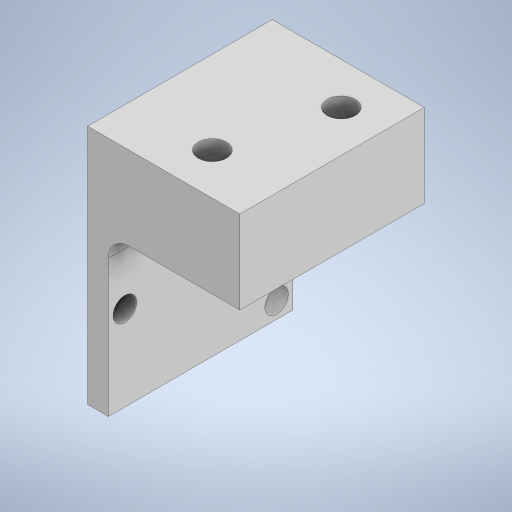
# Autodesk Inventor part: Limit Switch Top V1
Saved by Autodesk Inventor 2024.2 (Build 282272000, 272)
## iProperties
Created: 2024-08-22
Part Number: Limit Switch Top V1
Material: Generic
Document SubType Name: Modeling
Designer: balmo
Density: 1 g/cm^3
Appearance: Default
Author: balmo
## iProperties of the stored document Limit Switch Top V1_3DPrint.ipt
Created: 2024-08-22
Part Number: Limit Switch Top V1_3DPrint
Material: Generic
Document SubType Name: Modeling
Designer: balmo
Density: 1 g/cm^3
Appearance: Default
Author: balmo
Autodesk Inventor part; units mm, degrees
ref_plane "YZ Plane" through (0, 0, 0) normal (1, 0, 0) x (0, 1, 0)
ref_plane "XZ Plane" through (0, 0, 0) normal (0, 1, 0) x (-1, 0, 0)
ref_plane "XY Plane" through (0, 0, 0) normal (0, 0, 1) x (1, 0, 0)
sketch "Sketch1" plane through (0, 0, 0) normal (0, 0, 1) x (1, 0, 0)
  line L0 (0, 0) -> (3.175, 0)
  line L1 (3.175, 0) -> (3.175, 24.13)
  line L2 (0, 36.83) -> (0, 0)
  line L3 (23.2455, 36.83) -> (23.2455, 24.13)
  line L4 (23.2455, 24.13) -> (3.175, 24.13)
  line L5 (0, 36.83) -> (23.2455, 36.83)
  dimension "d0" = 12.7
  dimension "d1" = 3.175
  dimension "d2" = 36.83
  constraints: 12 end point, 2 horizontal, 1 parallel, 1 perpendicular
  measures "d0" distance between parallel lines of L4 L5
  measures "d1" distance between parallel lines of L2 L1
  measures "d2" distance between parallel lines of L5 L0
extrude "Extrusion1" add sketch "Sketch1" along normal blind 28.194
sketch "Sketch2" plane through (3.175, 0, 0) normal (1, 0, 0) x (0, 0, -1)
  circle A0 centre (-2.5, 2.5) radius 1.8
  circle A1 centre (-25.694, 13) radius 1.8
  line L0 (0, 0) -> (0, 24.13) projected
  line L1 (0, 0) -> (-28.194, 0) projected
  line L2 (-28.194, 0) -> (-28.194, 24.13) projected
  dimension "d5" = 3.6
  dimension "d6" = 3.6
  dimension "d7" = 2.5
  dimension "d8" = 2.5
  dimension "d9" = 2.5
  dimension "d10" = 13
  constraints: 2 centre point
  measures "d5" diameter of A0
  measures "d6" diameter of A1
  measures "d7" distance from line of A0.centre L0
  measures "d8" distance from line of A0.centre L1
  measures "d9" distance from line of L2 A1.centre
  measures "d10" distance from line of L1 A1.centre
extrude "Extrusion2" cut sketch "Sketch2" against normal blind 28.194
fillet "Fillet1" radius 3.175 1 edges at (3.175, 24.13, 14.097)
sketch "Sketch3" plane through (23.2455, 24.13, 0) normal (0, -1, 0) x (1, 0, 0)
  line L0 (-16.8955, 0) -> (-16.8955, 28.194) projected
  line L1 (-16.8955, 0) -> (0, 0) projected
  line L2 (0, 0) -> (0, 28.194) projected
  line L3 (-16.8955, 28.194) -> (0, 28.194) projected
  circle A0 centre (-10.5455, 21.844) radius 2.159
  circle A1 centre (-6.35, 6.35) radius 2.159
  point P0 (-23.2455, 0)
  dimension "d14" = 4.318
  dimension "d15" = 4.318
  dimension "d16" = 6.35
  dimension "d18" = 6.35
  dimension "d19" = 6.35
  dimension "d20" = 6.35
  constraints: 2 centre point
  measures "d14" diameter of A0
  measures "d15" diameter of A1
  measures "d16" distance from line of A1.centre L2
  measures "d18" distance from line of A1.centre L1
  measures "d19" distance from line of L3 A0.centre
  measures "d20" distance from line of A0.centre L0
extrude "Extrusion3" cut sketch "Sketch3" against normal blind 28.194 contours A0 | A1
chamfer "Chamfer1" distance 3.175 angle 45 2 edges at (14.7365, 24.13, 6.35) (10.541, 24.13, 21.844)
body "Solid1"
